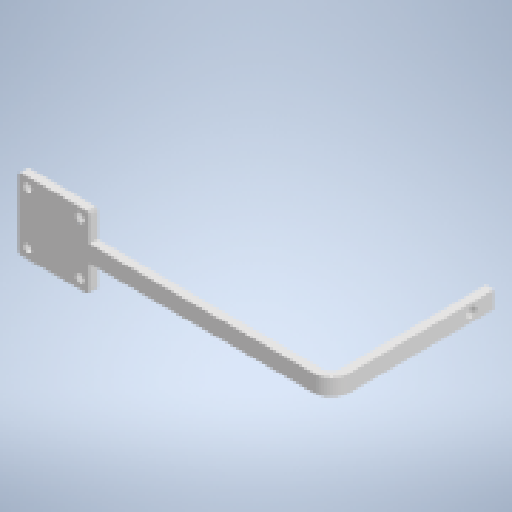
# Autodesk Inventor part: detenedor
Saved by Autodesk Inventor 2023 (Build 270158000, 158)
## iProperties
Created: 2023-03-05
Part Number: detenedor
Material: Generic
Document SubType Name: Sheet Metal
Designer: angel
Density: 1 g/cm^3
Sheet Metal Rule: Default_mm
Appearance: Default
Author: angel
Autodesk Inventor part; units mm, degrees
ref_plane "YZ Plane" through (0, 0, 0) normal (1, 0, 0) x (0, 1, 0)
ref_plane "XZ Plane" through (0, 0, 0) normal (0, 1, 0) x (-1, 0, 0)
ref_plane "XY Plane" through (0, 0, 0) normal (0, 0, 1) x (1, 0, 0)
sketch "Sketch1" plane through (0, 0, 0) normal (0, 0, 1) x (1, 0, 0)
  line L0 (-21.15, 19.15) -> (-21.15, -19.15)
  line L1 (21.15, -19.15) -> (21.15, 19.15)
  line L2 (19.15, 21.15) -> (-19.15, 21.15)
  line L3 (-19.15, -21.15) -> (19.15, -21.15)
  circle A0 centre (15.5, -15.5) radius 2.55
  circle A1 centre (15.5, 15.5) radius 2.55
  circle A2 centre (-15.5, 15.5) radius 2.55
  circle A3 centre (-15.5, -15.5) radius 2.55
  line L4 (-21.15, -19.15) -> (-21.15, 19.15)
  line L5 (-19.15, 21.15) -> (19.15, 21.15)
  line L6 (21.15, 19.15) -> (21.15, -19.15)
  line L7 (19.15, -21.15) -> (-19.15, -21.15)
  arc A4 (-21.15, -19.15) -> (-19.15, -21.15) centre (-19.15, -19.15) ccw
  arc A5 (-19.15, 21.15) -> (-21.15, 19.15) centre (-19.15, 19.15) ccw
  arc A6 (21.15, 19.15) -> (19.15, 21.15) centre (19.15, 19.15) ccw
  arc A7 (19.15, -21.15) -> (21.15, -19.15) centre (19.15, -19.15) ccw
  circle A8 centre (15.5, -15.5) radius 2.55
  circle A9 centre (15.5, 15.5) radius 2.55
  circle A10 centre (-15.5, 15.5) radius 2.55
  circle A11 centre (-15.5, -15.5) radius 2.55
  line L8 (159.3629, 5) -> (159.3629, -5)
  line L9 (138.2729, 5) -> (159.3629, 5)
  line L10 (159.3629, -5) -> (138.2729, -5)
  line L11 (21.15, -5) -> (159.3629, -5)
  line L12 (21.15, 5) -> (159.3629, 5)
  line L13 (159.3629, -5) -> (159.3629, 5)
  point P0 (0, 0)
  dimension "d0" = 2
  dimension "d1" = 10
  dimension "d2" = 5
  measures "d0" radius of A4
  measures "d1" distance between parallel lines of L12 L11
  measures "d2" distance from line of L12 point (0, 0)
sketch "Sketch2" plane through (159.3629, -5, 0) normal (1, 0, 0) x (0, 0, -1)
  line L0 (91.2, 10) -> (91.2, 0)
  line L1 (0, 10) -> (-5, 10)
  line L2 (-5, 10) -> (-5, 0)
  line L3 (0, 0) -> (-5, 0)
  line L4 (0, 10) -> (-5, 10)
  line L5 (-5, 10) -> (91.2, 10)
  line L6 (0, 0) -> (-5, 0)
  line L7 (-5, 0) -> (91.2, 0)
  line L8 (-5, 24.15) -> (-5, 10)
  line L9 (-5, 10) -> (-5, 0)
  line L10 (91.2, 10) -> (91.2, 0)
  circle A0 centre (78.1, 5) radius 2.75
  point P0 (0, 5)
  point P1 (78.1, 7.0932)
  point P2 (91.2, 5)
  dimension "d4" = 5.5
  measures "d4" diameter of A0
extrude "Plate1" add sketch "Sketch1" along normal blind 5
sheet face with bend "Face2" sketch "Sketch2" thickness 5 toward (1, 0, 0) bend radius 5
bend "Bend1"
equation "\"d3\" = Thickness"
equation "\"d5\" = BendRadius"
equation "\"d6\" = BendReliefWidth"
equation "\"d8\" = MinimumRemnant"
equation "\"d7\" = BendReliefDepth"
equation "\"d9\" = TransitionRadius"
equation "\"BendRadius\" = Thickness"
equation "\"BendReliefWidth\" = Thickness"
equation "\"BendReliefDepth\" = 0.5 * Thickness"
equation "\"TransitionRadius\" = BendRadius"
equation "\"JacobiRadiusSize\" = BendRadius"
equation "\"GapSize\" = Thickness"
equation "\"Thickness\" = 5"
equation "\"MinimumRemnant\" = 10"
body "Solid1"
